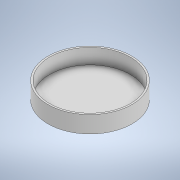
# Autodesk Inventor part: filterBase
Saved by Autodesk Inventor 2021 (Build 250183000, 183)
## iProperties
Created: 2020-04-12
Part Number: filterBase
Material: Generic
Document SubType Name: Modeling
Designer: robst
Density: 1 g/cm^3
Appearance: Default
Author: robst
Autodesk Inventor part; units mm, degrees
ref_plane "YZ Plane" through (0, 0, 0) normal (1, 0, 0) x (0, 1, 0)
ref_plane "XZ Plane" through (0, 0, 0) normal (0, 1, 0) x (-1, 0, 0)
ref_plane "XY Plane" through (0, 0, 0) normal (0, 0, 1) x (1, 0, 0)
sketch "Sketch3" plane through (0, 0, 0) normal (0, 0, 1) x (1, 0, 0)
  line L0 (0, 0) -> (63.5, 0)
  line L1 (63.5, 0) -> (63.5, 25.4)
  line L2 (63.5, 25.4) -> (60.96, 25.4)
  line L3 (60.96, 25.4) -> (60.96, 2.54)
  line L4 (60.96, 2.54) -> (0, 2.54)
  line L5 (0, 2.54) -> (0, 0)
  dimension "d3" = 63.5
  dimension "d4" = 25.4
  dimension "d5" = 2.54
  dimension "d6" = 22.86
  constraints: 12 end point, 3 perpendicular, 2 horizontal, 1 parallel
  measures "d3" distance of L0.start L0.end
  measures "d4" distance of L0.end L1.end
  measures "d5" distance of L1.end L2.end
  measures "d6" distance of L2.end L3.end
revolve "Revolution1" add sketch "Sketch3" angle 360 about axis through (0, 2.54, 0) along (0, -1, 0)
body "Solid2"
